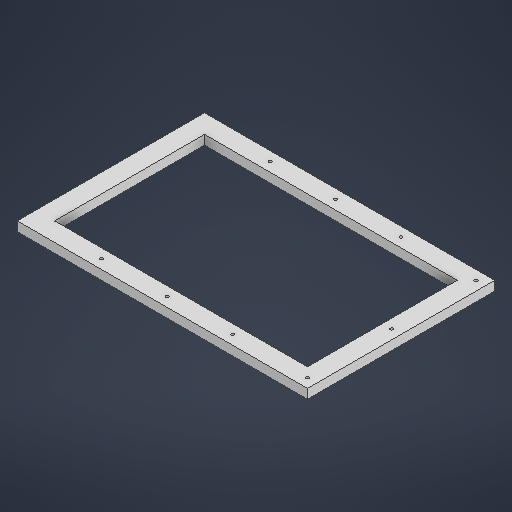
# Autodesk Inventor part: Aufhängung_Seitenteil_Koppeltest_außen
Saved by Autodesk Inventor 2027 (Build 310192060, 192F)
## iProperties
Created: 2026-07-21
Part Number: Aufhängung_Seitenteil_Koppeltest_außen
Material: Generic
Document SubType Name: Modeling
Designer: kw
Density: 1 g/cm^3
Appearance: Default
Author: kw
Autodesk Inventor part; units mm, degrees
ref_plane "YZ Plane" through (0, 0, 0) normal (1, 0, 0) x (0, 1, 0)
ref_plane "XZ Plane" through (0, 0, 0) normal (0, 1, 0) x (-1, 0, 0)
ref_plane "XY Plane" through (0, 0, 0) normal (0, 0, 1) x (1, 0, 0)
sketch "Sketch1" plane through (0, 0, 0) normal (0, 1, 0) x (-1, 0, 0)
  line L0 (100, -400) -> (-100, -400)
  line L1 (-100, -400) -> (-100, -110)
  line L2 (-100, -110) -> (100, -110)
  line L3 (100, -400) -> (100, -110)
  line L4 (100, -110) -> (100, -400)
  line L5 (-100, -90) -> (100, -90)
  line L6 (100, -110) -> (100, -90)
  line L7 (-100, -110) -> (-100, -90)
  line L8 (-80, -390) -> (-80, -110)
  line L9 (80, -390) -> (80, -110)
  line L10 (-80, -380) -> (80, -380)
  point P0 (0, -100)
  point P1 (90, -100)
  point P2 (-90, -100)
  dimension "d126" = 160
  dimension "d160" = 290
  constraints: 22 end point, 4 perpendicular, 4 point on line, 2 vertical, 1 parallel
  measures "d126" distance of L9.start L8.start
  measures "d160" distance of L0.end L1.end
extrude "Extrusion1" add sketch "Sketch1" along normal blind 10 contours L0 L1 L2 L8 L10 L9 L3 | L2 L7 L5 L6
sketch "Sketch12" plane through (0, 10, 0) normal (0, 1, 0) x (1, 0, 0)
  line L0 (90, 400) -> (90, 320)
  line L1 (90, 320) -> (90, 250)
  line L2 (90, 250) -> (90, 180)
  point P0 (0, 0)
  dimension "d132" = 80
  dimension "d134" = 70
  dimension "d135" = 70
  constraints: 6 end point, 2 point on line, 1 vertical
  measures "d132" distance of L0.start L0.end
  measures "d134" distance of L0.end L1.end
  measures "d135" distance of L1.end L2.end
hole "Hole9" at (90, 10, -320) at (90, 10, -250) at (90, 10, -180) direction (0, -1, 0) diameter 3.2 end through all clearance for "Socket Head Cap Screw ISO 4762" size "M3" standard "ISO"
pattern_linear "Rectangular Pattern1" count 2 spacing 180 along (-1, 0, 0) of "Hole9"
hole "Hole12" at (90, 0, -100) at (-90, 0, -100) direction (0, 1, 0) diameter 3.4 end through all clearance for "Socket Head Cap Screw ISO 4762" size "M3" standard "ISO"
hole "Hole13" at (0, 0, -100) direction (0, 1, 0) diameter 3 end through all
body "Solid1"
